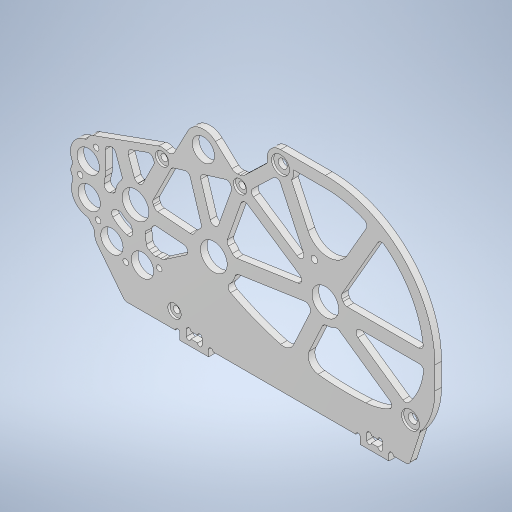
# Autodesk Inventor part: ギアマウント
Saved by Autodesk Inventor 2023 (Build 270158000, 158)
## iProperties
Created: 2022-03-20
Part Number: ギアマウント
Material: Aluminum 2014-T6
Document SubType Name: Modeling
Designer: acps
Density: 2.78927 g/cm^3
Appearance: Satin
Author: acps
Autodesk Inventor part; units mm, degrees
ref_plane "YZ Plane" through (0, 0, 0) normal (1, 0, 0) x (0, 1, 0)
ref_plane "XZ Plane" through (0, 0, 0) normal (0, 1, 0) x (-1, 0, 0)
ref_plane "XY Plane" through (0, 0, 0) normal (0, 0, 1) x (1, 0, 0)
sketch "Sketch2" plane through (0, 0, 0) normal (0, 0, 1) x (1, 0, 0)
  line L0 (-44.2416, -60) -> (63.0185, -60) construction
  line L1 (-44.2416, -60) -> (63.0185, -60) construction
  circle A0 centre (-30.6992, 12) radius 14 construction
  circle A1 centre (-44.5148, 14.4973) radius 14 construction
  circle A2 centre (-50.7402, 19.5218) radius 1.25
  circle A3 centre (-38.2895, 9.4728) radius 1.25
  circle A4 centre (-23.1088, 14.5272) radius 1.25
  circle A5 centre (-58.8465, 33.3162) radius 1.25
  circle A6 centre (-51.6122, 47.5873) radius 1.25
  circle A7 centre (-55.2294, 40.4518) radius 14 construction
  circle A8 centre (-54.7933, 26.419) radius 14 construction
  circle A9 centre (-33.8392, 34.0933) radius 22.3153 construction
  circle A10 centre (1.5644, 31.4) radius 30.9859 construction
  circle A11 centre (52, 38.9589) radius 41.9589 construction
  circle A12 centre (-55.2294, 40.4518) radius 5.025
  arc A13 (-56.8528, 48.3109) -> (-62.589, 43.6511) centre (-55.2294, 40.4518) ccw
  circle A14 centre (-54.7933, 26.419) radius 5.025
  circle A15 centre (-54.7933, 26.419) radius 8.025
  circle A16 centre (-50.7402, 19.5218) radius 4.25 construction
  arc A17 (-36.8441, 5.4762) -> (-41.0426, 6.2351) centre (-38.2895, 9.4728) ccw construction
  arc A18 (-24.5543, 18.5238) -> (-21.87, 10.4617) centre (-23.1088, 14.5272) ccw construction
  circle A19 centre (-44.5148, 14.4973) radius 5.025
  circle A20 centre (-30.6992, 12) radius 5.025
  circle A21 centre (-44.5148, 14.4973) radius 8.025
  circle A22 centre (-30.6992, 12) radius 8.025
  arc A23 (-41.0426, 6.2351) -> (-42.7724, 6.6637) centre (-42.3382, 4.7114) ccw
  arc A24 (-56.8528, 48.3109) -> (-55.451, 49.4112) centre (-57.2574, 50.2695) ccw
  arc A25 (-35.0737, 5.2721) -> (-36.8441, 5.4762) centre (-36.1639, 3.5954) ccw
  circle A26 centre (-21.8397, 58.0739) radius 1.5
  circle A27 centre (-21.8397, 58.0739) radius 4.5
  circle A28 centre (13.4218, 64.8462) radius 1.5
  circle A29 centre (13.4218, 64.8462) radius 4.5
  circle A30 centre (31.7211, 82.4471) radius 6.025
  circle A31 centre (31.7211, 82.4471) radius 4.025
  circle A32 centre (90.487, 12.01) radius 5.025
  circle A33 centre (90.487, 12.01) radius 2.025
  line L2 (-53.0558, 51.5846) -> (-23.3682, 62.3063)
  arc A34 (-18.3854, 60.958) -> (-16.2563, 60.33) centre (-16.8502, 62.2398) ccw
  line L3 (-16.2563, 60.33) -> (12.0856, 69.1432)
  circle A35 centre (-33.8392, 34.0933) radius 6.025
  circle A36 centre (-33.8392, 34.0933) radius 9.025
  arc A37 (-47.4788, 38.3562) -> (-31.6308, 19.9746) centre (-33.8392, 34.0933) ccw
  line L4 (-46.0723, 50.9171) -> (-28.4446, 57.2833)
  arc A38 (-25.942, 56.2243) -> (-28.4446, 57.2833) centre (-27.7652, 55.4023) ccw
  arc A39 (-25.6321, 53.8469) -> (-25.7034, 55.7671) centre (-27.4207, 54.7419) ccw
  line L5 (-25.6321, 53.8469) -> (-30.5023, 44.114)
  arc A40 (-32.5717, 43.0288) -> (-30.5023, 44.114) centre (-32.2908, 45.009) ccw
  line L6 (-17.8154, 56.0602) -> (-25.8299, 40.0433)
  arc A41 (-25.8299, 40.0433) -> (-25.8187, 38.2313) centre (-24.0414, 39.1483) ccw
  line L7 (-33.8392, 34.0933) -> (-21.8397, 58.0739) construction
  line L8 (-47.4788, 38.3562) -> (-47.4212, 38.5991)
  line L9 (-47.2048, 40.5594) -> (-47.3924, 48.9915)
  arc A42 (-46.0723, 50.9171) -> (-47.3924, 48.9915) centre (-45.3929, 49.036) ccw
  line L10 (-54.7933, 26.419) -> (-33.8392, 34.0933) construction
  arc A43 (-48.0965, 35.0629) -> (-45.4133, 33.0492) centre (-46.1011, 34.9272) ccw
  arc A44 (-43.3499, 27.4152) -> (-44.0979, 24.1448) centre (-42.6621, 25.5372) ccw
  arc A45 (-44.0976, 33.5311) -> (-42.7997, 35.1704) centre (-44.7854, 35.4091) ccw
  arc A46 (-39.9845, 27.4838) -> (-42.0342, 27.8971) centre (-41.3464, 26.019) ccw
  line L11 (-45.4133, 33.0492) -> (-44.0976, 33.5311)
  line L12 (-43.3499, 27.4152) -> (-42.0342, 27.8971)
  line L13 (-33.8392, 34.0933) -> (-30.6992, 12) construction
  arc A47 (-35.4267, 23.9429) -> (-36.7596, 25.5538) centre (-37.4068, 23.6614) ccw
  arc A48 (-28.6551, 26.7057) -> (-29.4864, 24.7871) centre (-27.5063, 25.0686) ccw
  arc A49 (-37.7581, 20.3508) -> (-35.2295, 22.5556) centre (-37.2096, 22.2742) ccw
  arc A50 (-28.9517, 21.0248) -> (-27.7152, 19.4496) centre (-26.9716, 21.3062) ccw
  line L14 (-35.4267, 23.9429) -> (-35.2295, 22.5556)
  line L15 (-29.4864, 24.7871) -> (-28.9517, 21.0248)
  arc A51 (-42.7678, 49.9841) -> (-45.3282, 51.1858) centre (-44.6489, 49.3047) ccw
  arc A52 (-35.9228, 54.5826) -> (-37.1245, 52.0221) centre (-35.2435, 52.7015) ccw
  arc A53 (-40.421, 40.2682) -> (-39.9985, 42.316) centre (-41.8796, 41.6367) ccw
  arc A54 (-34.3552, 44.3541) -> (-32.7218, 43.0488) centre (-32.4741, 45.0334) ccw
  line L16 (-42.7678, 49.9841) -> (-39.9985, 42.316)
  line L17 (-34.3552, 44.3541) -> (-37.1245, 52.0221)
  line L18 (-33.8392, 34.0933) -> (-40.6255, 52.8842) construction
  circle A55 centre (1.5644, 31.4) radius 6.025
  circle A56 centre (52, 38.9589) radius 6.025
  circle A57 centre (1.5644, 31.4) radius 10.025
  circle A58 centre (52, 38.9589) radius 9.025
  arc A59 (-16.6207, 57.075) -> (-17.8154, 56.0602) centre (-16.0268, 55.1652) ccw
  line L19 (-16.6207, 57.075) -> (6.788, 64.3542)
  arc A60 (9.2403, 63.1834) -> (6.788, 64.3542) centre (7.3818, 62.4444) ccw
  arc A61 (-26.3247, 18.7279) -> (-24.5543, 18.5238) centre (-25.2345, 20.4046) ccw
  arc A62 (-21.87, 10.4617) -> (-23.1648, 9.2372) centre (-21.287, 8.5486) ccw
  arc A63 (-22.4016, 18.7179) -> (-20.9398, 19.0391) centre (-22.0688, 20.69) ccw
  arc A64 (-18.1174, 14.9119) -> (-18.947, 13.6662) centre (-16.9884, 13.261) ccw
  line L20 (-20.9398, 19.0391) -> (-11.0791, 25.7824)
  arc A65 (-9.0516, 27.1689) -> (-8.2271, 29.249) centre (-10.1805, 28.8198) ccw construction
  arc A66 (-3.9917, 23.0555) -> (-6.2292, 23.0417) centre (-5.1002, 21.3908) ccw
  line L21 (-18.1174, 14.9119) -> (-6.2292, 23.0417)
  line L22 (-23.1088, 14.5272) -> (1.5644, 31.4) construction
  arc A67 (-25.5084, 37.5643) -> (-23.8139, 36.3393) centre (-23.6622, 38.3335) ccw
  arc A68 (-24.269, 30.3566) -> (-26.1293, 29.4019) centre (-24.4207, 28.3623) ccw
  arc A69 (-9.1127, 35.2209) -> (-7.2104, 36.248) centre (-8.961, 37.2151) ccw
  arc A70 (-7.8428, 27.9352) -> (-9.5679, 29.2382) centre (-9.7196, 27.244) ccw construction
  line L23 (-23.8139, 36.3393) -> (-9.1127, 35.2209)
  line L24 (-24.269, 30.3566) -> (-12.0564, 29.4275)
  line L25 (-33.8392, 34.0933) -> (1.5644, 31.4) construction
  arc A71 (-11.0791, 25.7824) -> (-12.0564, 29.4275) centre (-12.2081, 27.4333) ccw
  line L26 (-12.0564, 29.4275) -> (-9.5679, 29.2382) construction
  line L27 (-11.0791, 25.7824) -> (-9.0516, 27.1689) construction
  line L28 (-7.319, 59.9675) -> (1.5644, 31.4) construction
  arc A72 (-9.1123, 57.3153) -> (-11.616, 58.6313) centre (-11.0221, 56.7215) ccw
  arc A73 (-3.0219, 61.3037) -> (-4.3379, 58.8) centre (-2.4281, 59.3939) ccw
  arc A74 (-4.7785, 39.1633) -> (-4.2408, 41.5776) centre (-6.0439, 40.7121) ccw
  arc A75 (0.6404, 42.7907) -> (2.3863, 41.3913) centre (2.5502, 43.3845) ccw construction
  line L29 (-9.1123, 57.3153) -> (-4.1341, 41.306)
  line L30 (-4.3379, 58.8) -> (-0.0658, 45.0619)
  arc A76 (-55.451, 49.4112) -> (-55.772, 48.4584) centre (-51.6122, 47.5873) ccw construction
  arc A77 (-55.772, 48.4584) -> (-56.8528, 48.3109) centre (-55.2294, 40.4518) ccw construction
  arc A78 (-62.589, 43.6511) -> (-62.0081, 36.1565) centre (-55.2294, 40.4518) ccw
  arc A79 (-62.0081, 36.1565) -> (-55.772, 48.4584) centre (-55.2294, 40.4518) ccw
  arc A80 (-53.0558, 51.5846) -> (-55.451, 49.4112) centre (-51.6122, 47.5873) ccw
  arc A81 (-41.0426, 6.2351) -> (-36.8441, 5.4762) centre (-38.2895, 9.4728) ccw
  arc A82 (-22.4016, 18.7179) -> (-24.5543, 18.5238) centre (-23.1088, 14.5272) ccw
  arc A83 (-18.947, 13.6662) -> (-22.4016, 18.7179) centre (-23.1088, 14.5272) ccw construction
  arc A84 (-21.4252, 10.6249) -> (-18.947, 13.6662) centre (-23.1088, 14.5272) ccw
  arc A85 (-21.87, 10.4617) -> (-21.4252, 10.6249) centre (-23.1088, 14.5272) ccw
  arc A86 (9.9632, 36.8737) -> (11.9352, 35.9878) centre (11.6387, 37.9657) ccw
  arc A87 (12.8245, 30.0541) -> (11.1988, 28.629) centre (13.1209, 28.0762) ccw
  arc A88 (41.8379, 40.4694) -> (43.4387, 41.8145) centre (41.5414, 42.4473) ccw construction
  arc A89 (44.652, 33.7189) -> (42.7272, 34.5357) centre (43.0236, 32.5577) ccw
  line L31 (11.9352, 35.9878) -> (39.536, 40.1244)
  line L32 (12.8245, 30.0541) -> (42.7272, 34.5357)
  line L33 (1.5644, 31.4) -> (52, 38.9589) construction
  arc A90 (9.4982, 61.2607) -> (9.4005, 62.8266) centre (7.6132, 61.929) ccw
  arc A91 (15.2731, 60.7446) -> (14.2108, 59.59) centre (16.0959, 58.9217) ccw construction
  arc A92 (1.1349, 41.4158) -> (2.9342, 42.7457) centre (1.0492, 43.414) ccw construction
  arc A93 (7.6468, 41.0749) -> (8.2067, 38.9087) centre (9.5319, 40.4067) ccw
  line L34 (2.9342, 42.7457) -> (3.729, 44.9875) construction
  line L35 (14.2108, 59.59) -> (13.8416, 58.5486) construction
  line L36 (1.5644, 31.4) -> (13.4218, 64.8462) construction
  arc A94 (-0.0658, 45.0619) -> (3.729, 44.9875) centre (1.844, 45.6558) ccw
  line L37 (-0.0658, 45.0619) -> (0.6404, 42.7907) construction
  line L38 (3.729, 44.9875) -> (9.4982, 61.2607)
  line L39 (13.4218, 64.8462) -> (52, 38.9589) construction
  arc A95 (15.9236, 60.1567) -> (14.3823, 60.4499) centre (14.8092, 58.496) ccw construction
  arc A96 (17.8541, 65.6237) -> (18.7096, 64.3086) centre (19.824, 65.9693) ccw construction
  arc A97 (43.106, 40.4909) -> (42.2494, 42.4912) centre (41.135, 40.8304) ccw construction
  arc A98 (45.0355, 46.643) -> (47.2111, 46.6086) centre (46.1499, 48.3038) ccw construction
  line L40 (18.7096, 64.3086) -> (19.45, 63.8118) construction
  line L41 (42.2494, 42.4912) -> (40.354, 43.7631) construction
  arc A99 (16.8411, 59.541) -> (13.8416, 58.5486) centre (15.7267, 57.8803) ccw
  line L42 (13.8416, 58.5486) -> (7.6468, 41.0749)
  line L43 (16.8411, 59.541) -> (15.9236, 60.1567) construction
  arc A100 (39.536, 40.1244) -> (40.354, 43.7631) centre (39.2396, 42.1023) ccw
  line L44 (40.354, 43.7631) -> (16.8411, 59.541)
  line L45 (39.536, 40.1244) -> (41.8379, 40.4694) construction
  line L46 (31.7211, 82.4471) -> (52, 38.9589) construction
  line L47 (52, 38.9589) -> (90.487, 12.01) construction
  line L48 (52, 38.9589) -> (96.5132, 38.9589) construction
  arc A101 (-3.9917, 23.0555) -> (91.7705, 7.1517) centre (61.5599, 121.5041) ccw
  arc A102 (9.1166, 21.0995) -> (70.407, 8.5744) centre (61.5599, 121.5041) ccw
  arc A103 (8.6324, 24.2906) -> (9.1166, 21.0995) centre (10.0425, 22.8723) ccw
  arc A104 (45.1595, 31.2935) -> (44.9138, 33.3699) centre (43.3435, 32.1314) ccw
  arc A105 (52.3468, 29.9406) -> (50.6076, 28.7799) centre (52.4236, 27.942) ccw
  line L49 (45.1595, 31.2935) -> (37.6177, 14.9471)
  line L50 (50.6076, 28.7799) -> (44.7222, 16.0237)
  arc A106 (31.7623, 12.2178) -> (37.6177, 14.9471) centre (33.0776, 17.0418) ccw
  arc A107 (44.7222, 16.0237) -> (48.6944, 8.9614) centre (49.2623, 13.929) ccw
  line L51 (38.88, 10.5221) -> (52, 38.9589) construction
  arc A108 (13.6025, 69.3426) -> (15.0693, 69.8995) centre (13.6828, 71.341) ccw
  arc A109 (18.5354, 66.2959) -> (17.9218, 64.8519) centre (19.9218, 64.8544) ccw construction
  line L52 (15.0693, 69.8995) -> (25.1991, 79.6427)
  arc A110 (25.1991, 79.6427) -> (25.7837, 81.4239) centre (23.8127, 81.0842) ccw
  arc A111 (30.4677, 76.5539) -> (28.6652, 76.0391) centre (30.0517, 74.5976) ccw construction
  line L53 (18.5354, 66.2959) -> (19.178, 66.914) construction
  line L54 (13.4218, 64.8462) -> (31.7211, 82.4471) construction
  arc A112 (19.178, 66.914) -> (19.45, 63.8118) centre (20.5644, 65.4725) ccw
  line L55 (19.178, 66.914) -> (28.536, 75.9148)
  line L56 (19.45, 63.8118) -> (39.1784, 50.5734)
  arc A113 (31.655, 75.4903) -> (30.3106, 76.5895) centre (29.8424, 74.6451) ccw construction
  arc A114 (44.8912, 44.519) -> (45.1284, 46.5964) centre (43.3158, 45.7512) ccw construction
  line L57 (45.1284, 46.5964) -> (42.1054, 53.0793) construction
  arc A115 (37.115, 79.7624) -> (37.0928, 78.026) centre (38.9054, 78.8713) ccw construction
  line L58 (44.165, 62.8598) -> (35.8801, 80.6268)
  arc A116 (31.7351, 75.3186) -> (28.536, 75.9148) centre (29.9224, 74.4734) ccw
  line L59 (28.536, 75.9148) -> (28.6652, 76.0391) construction
  line L60 (31.7351, 75.3186) -> (31.655, 75.4903) construction
  arc A117 (39.1784, 50.5734) -> (42.1054, 53.0793) centre (40.2928, 52.2341) ccw
  line L61 (42.1054, 53.0793) -> (31.7351, 75.3186)
  line L62 (39.1784, 50.5734) -> (45.0355, 46.643) construction
  arc A118 (101.5132, 38.9589) -> (52, 88.4721) centre (52, 38.9589) ccw
  arc A119 (39.6867, 83.4721) -> (37.7015, 81.7151) centre (39.6867, 81.4721) ccw construction
  line L63 (31.7211, 88.4721) -> (52, 88.4721)
  line L64 (39.6867, 83.4721) -> (37.6927, 83.4721) construction
  arc A120 (37.6927, 83.4721) -> (35.8801, 80.6268) centre (37.6927, 81.4721) ccw
  line L65 (37.6927, 83.4721) -> (52, 83.4721)
  line L66 (35.8801, 80.6268) -> (37.0928, 78.026) construction
  arc A121 (96.5132, 38.9589) -> (52, 83.4721) centre (52, 38.9589) ccw
  line L67 (96.5132, 38.9589) -> (96.5132, 36.8058)
  line L68 (101.5132, 38.9589) -> (101.5132, 28.7597)
  arc A122 (94.3686, 8.8189) -> (101.5132, 28.7597) centre (70.1132, 28.7597) ccw
  arc A123 (70.407, 8.5744) -> (96.5132, 36.8058) centre (68.1953, 36.8058) ccw
  arc A124 (58.3283, 30.8655) -> (56.2412, 30.9926) centre (57.1811, 29.2272) ccw
  arc A125 (60.9365, 37.6981) -> (61.7697, 35.7804) centre (62.9169, 37.4187) ccw
  arc A126 (80.866, 11.4808) -> (81.1183, 14.9077) centre (79.9711, 13.2694) ccw
  arc A127 (87.0584, 18.0731) -> (89.7262, 18.4123) centre (88.2056, 19.7114) ccw
  line L69 (58.3283, 30.8655) -> (81.1183, 14.9077)
  line L70 (61.7697, 35.7804) -> (87.0584, 18.0731)
  line L71 (52, 38.9589) -> (74.2566, 77.5084) construction
  arc A128 (59.5111, 45.9685) -> (59.5664, 43.8783) centre (61.2431, 44.9685) ccw
  arc A129 (70.511, 77.0209) -> (69.5683, 79.8585) centre (68.7789, 78.0209) ccw
  arc A130 (78.636, 74.6233) -> (75.7071, 74.0209) centre (77.4392, 73.0209) ccw
  line L72 (70.511, 77.0209) -> (61.8883, 62.0859)
  line L73 (59.5111, 45.9685) -> (75.7071, 74.0209)
  line L74 (61.826, 41.9589) -> (94.2181, 41.9589)
  line L75 (67.858, 35.9589) -> (94.5132, 35.9589)
  arc A131 (67.858, 35.9589) -> (66.7108, 32.3206) centre (67.858, 33.9589) ccw
  arc A132 (60.0435, 43.0519) -> (61.826, 41.9589) centre (61.826, 43.9589) ccw
  arc A133 (94.2181, 41.9589) -> (96.2042, 44.1941) centre (94.2181, 43.9589) ccw
  arc A134 (96.5132, 33.9589) -> (94.5132, 35.9589) centre (94.5132, 33.9589) ccw
  arc A135 (-39.285, -5.2313) -> (-37.709, -6) centre (-37.709, -4) ccw
  line L76 (-33.8392, 34.0933) -> (-16.1374, 34.0933) construction
  line L77 (1.5644, 34.0933) -> (1.5644, 31.4) construction
  line L78 (-16.1374, 34.0933) -> (-16.1374, 29.0871) construction
  arc A136 (88.4657, -6) -> (90.3678, -4.618) centre (88.4657, -4) ccw
  arc A137 (-62.5868, 35.3343) -> (-62.528, 37.1155) centre (-64.347, 36.284) ccw
  arc A138 (-62.5868, 35.3343) -> (-62.4543, 31.0698) centre (-58.8465, 33.3162) ccw
  arc A139 (-62.285, 29.2957) -> (-62.4543, 31.0698) centre (-64.1521, 30.0127) ccw
  line L79 (-37.709, -6) -> (88.4657, -6)
  line L80 (-10.7865, -3) -> (77.7566, -3)
  circle A140 centre (-9.7865, -3) radius 1
  circle A141 centre (-4.7865, -3) radius 1
  circle A142 centre (-9.7865, -6) radius 1
  circle A143 centre (-4.7865, -6) radius 1
  line L81 (-10.7865, -3) -> (-10.7865, -6)
  line L82 (-3.7865, -3) -> (-3.7865, -6)
  circle A144 centre (-14.7865, -6) radius 1
  circle A145 centre (0.2135, -6) radius 1
  circle A146 centre (71.7566, -3) radius 1
  circle A147 centre (76.7566, -3) radius 1
  circle A148 centre (71.7566, -6) radius 1
  circle A149 centre (76.7566, -6) radius 1
  line L83 (77.7566, -3) -> (77.7566, -6)
  line L84 (70.7566, -3) -> (70.7566, -6)
  circle A150 centre (66.7566, -6) radius 1
  circle A151 centre (81.7566, -6) radius 1
  line L85 (-13.7865, -6) -> (-13.7865, -9)
  line L86 (-13.7865, -9) -> (-0.7865, -9)
  line L87 (-0.7865, -9) -> (-0.7865, -6)
  line L88 (67.7566, -6) -> (67.7566, -9)
  line L89 (67.7566, -9) -> (80.7566, -9)
  line L90 (80.7566, -9) -> (80.7566, -6)
  circle A152 centre (-16.2379, 1.2821) radius 1.5
  circle A153 centre (-16.2379, 1.2821) radius 3
  circle A154 centre (-16.2379, 1.2821) radius 4 construction
  arc A155 (-54.4583, 17.4631) -> (-55.9258, 18.4743) centre (-56.208, 16.4943) ccw
  arc A156 (-54.4583, 17.4631) -> (-53.3238, 16.1473) centre (-50.7402, 19.5218) ccw
  arc A157 (-52.5397, 14.5469) -> (-53.3238, 16.1473) centre (-54.5396, 14.5593) ccw
  line L91 (-39.285, -5.2313) -> (-50.8386, 9.5566)
  line L92 (-16.1374, 34.0933) -> (1.5644, 34.0933) construction
  line L93 (-7.2865, 34.0933) -> (-7.2865, -12.1424) construction
  circle A158 centre (-21.8397, 58.0739) radius 3
  circle A159 centre (13.4218, 64.8462) radius 3
  circle A160 centre (-3.14, 71) radius 5.025
  circle A161 centre (-3.14, 71) radius 8.025
  line L94 (-10.2436, 74.7336) -> (-16.1326, 63.5293)
  arc A162 (-20.0087, 62.1846) -> (-16.1326, 63.5293) centre (-18.7881, 64.925) ccw
  line L95 (2.3049, 76.8952) -> (9.7999, 69.9727)
  arc A163 (9.7999, 69.9727) -> (12.4699, 69.2444) centre (11.8354, 72.1765) ccw
  line L96 (95.266, 10.4572) -> (90.3678, -4.618)
  line L97 (74.2566, 38.9589) -> (74.2566, -10.9885) construction
  circle A164 centre (31.7211, 82.4471) radius 2.025
  circle A165 centre (47, 53.101) radius 1.5
  arc A166 (44.165, 62.8598) -> (61.8883, 62.0859) centre (53.2281, 67.0859) ccw
  circle A167 centre (90.487, 12.01) radius 4.025
  point P0 (0, 0)
  point P1 (-47.2064, 40.6303)
  point P2 (-47.537, 38.1651)
  point P3 (96.4233, 34.5517)
  point P4 (36.6482, 78.9795)
  point P5 (37.6584, 83.4718)
  point P6 (72.7566, -3)
  point P7 (75.7566, -3)
  point P8 (75.7566, -6)
  point P9 (72.7566, -6)
  point P10 (-5.7865, -6)
  point P11 (-8.7865, -6)
  point P12 (-8.7865, -3)
  point P13 (-5.7865, -3)
  point P14 (-15.7865, -6)
  point P15 (1.2135, -6)
  point P16 (65.7566, -6)
  point P17 (82.7566, -6)
  point P18 (94.9855, 9.5939)
  dimension "d1136" = 2
  dimension "d1137" = 2
  dimension "d1139" = 2
  dimension "d1140" = 2
  dimension "d1142" = 2
  dimension "d1144" = 2
  dimension "d1146" = 2
  dimension "d1147" = 2
  dimension "d1149" = 2
  dimension "d1150" = 2
  dimension "d1152" = 2
  dimension "d1153" = 2
  dimension "d984" = 60
  dimension "d985" = 10.05
  dimension "d986" = 3
  dimension "d987" = 10.05
  dimension "d988" = 3
  dimension "d989" = 3
  dimension "d990" = 3
  dimension "d991" = 3
  dimension "d992" = 10.05
  dimension "d993" = 10.05
  dimension "d994" = 3
  dimension "d995" = 3
  dimension "d996" = 2
  dimension "d997" = 2
  dimension "d998" = 2
  dimension "d999" = 3
  dimension "d1000" = 3
  dimension "d1001" = 3
  dimension "d1002" = 3
  dimension "d1003" = 8.05
  dimension "d1004" = 2
  dimension "d1005" = 4.05
  dimension "d1006" = 3
  dimension "d1007" = 2
  dimension "d1008" = 12.05
  dimension "d1009" = 3
  dimension "d1010" = 2
  dimension "d1011" = 3
  dimension "d1012" = 2
  dimension "d1013" = 2
  dimension "d1014" = 2
  dimension "d1015" = 6
  dimension "d1016" = 2
  dimension "d1017" = 2
  dimension "d1018" = 2
  dimension "d1019" = 2
  dimension "d1020" = 2
  dimension "d1021" = 3
  dimension "d1022" = 6
  dimension "d1023" = 2
  dimension "d1024" = 2
  dimension "d1025" = 2
  dimension "d1026" = 2
  dimension "d1027" = 6
  dimension "d1028" = 3
  dimension "d1029" = 2
  dimension "d1030" = 2
  dimension "d1031" = 2
  dimension "d1032" = 2
  dimension "d1033" = 6
  dimension "d1034" = 3
  dimension "d1035" = 12.05
  dimension "d1036" = 12.05
  dimension "d1037" = 4
  dimension "d1038" = 3
  dimension "d1039" = 2
  dimension "d1040" = 2
  dimension "d1041" = 3
  dimension "d1042" = 2
  dimension "d1043" = 2
  dimension "d1044" = 2
  dimension "d1045" = 2
  dimension "d1046" = 2
  dimension "d1047" = 2
  constraints: 266 point on circle, 217 tangent, 194 end point, 148 centre point, 60 parallel, 14 point on line, 14 vertical, 13 coincident, 9 horizontal, 7 perpendicular, 5 concentric, 2 midpoint, 192 other
  measures "d984" distance from line of L1 point (0, 0)
  measures "d985" diameter of A12
  measures "d987" diameter of A14
  measures "d988" radial gap between concentric circles of A14 A15
  measures "d989" radial gap between concentric circles of A2 A16
  measures "d990" radial gap between concentric circles of A3 A17
  measures "d991" radial gap between concentric circles of A4 A18
  measures "d992" diameter of A19
  measures "d993" diameter of A20
  measures "d994" radial gap between concentric circles of A19 A21
  measures "d995" radial gap between concentric circles of A20 A22
  measures "d996" radius of A24
  measures "d997" radius of A23
  measures "d998" radius of A25
  measures "d999" diameter of A26
  measures "d1000" radial gap between concentric circles of A26 A27
  measures "d1001" diameter of A28
  measures "d1002" diameter of A28
  measures "d1003" diameter of A31
  measures "d1004" radial gap between concentric circles of A31 A30
  measures "d1005" diameter of A33
  measures "d1006" radial gap between concentric circles of A33 A32
  measures "d1007" radius of A34
  measures "d1008" diameter of A35
  measures "d1010" radius of A38
  measures "d1011" distance between parallel lines of L2 L4
  measures "d1012" radius of A39
  measures "d1013" radius of A40
  measures "d1014" radius of A41
  measures "d1015" distance between parallel lines of L5 L6
  measures "d1016" radius of A42
  measures "d1017" radius of A43
  measures "d1018" radius of A44
  measures "d1019" radius of A45
  measures "d1020" radius of A46
  measures "d1021" distance between parallel lines of L11 L10
  measures "d1022" distance between parallel lines of L12 L11
  measures "d1023" radius of A47
  measures "d1024" radius of A48
  measures "d1025" radius of A49
  measures "d1026" radius of A50
  measures "d1027" distance between parallel lines of L15 L14
  measures "d1028" distance between parallel lines of L14 L13
  measures "d1029" radius of A51
  measures "d1030" radius of A52
  measures "d1031" radius of A53
  measures "d1032" radius of A54
  measures "d1033" distance between parallel lines of L17 L16
  measures "d1034" distance between parallel lines of L16 L18
  measures "d1035" diameter of A55
  measures "d1036" diameter of A56
  measures "d1039" radius of A59
  measures "d1040" radius of A60
  measures "d1041" distance between parallel lines of L19 L3
  measures "d1042" radius of A61
  measures "d1043" radius of A62
  measures "d1044" radius of A63
  measures "d1045" radius of A64
  measures "d1046" radius of A65
  measures "d1047" radius of A66
extrude "Extrusion1" add sketch "Sketch2" along normal blind 3 contours A2 A15 A21 A22 A3 | A2 A21 A15 | A21 A157 A156 A155 A15 A2 | A2 A15 A5 A79 A21 | A15 A37 A21 | A37 A22 A21 | A21 A23 A81 A25 A22 A62 A85 A84 A64 L21 A66 A101 A32 A122 L96 A136 L79 A151 L83 A147 L80 A146 A141 A140 L81 A144 A135 L91 | A15 A79 A37 | A37 A43 L11 A45 A36 A46 L12 A44 | A22 A4 A3 A21 | A21 A3 A22 | A49 L14 A47 A36 A48 L15 A50 A22 A37 | A139 A138 A137 A78 A79 A5 A15 | A21 A3 A22 A25 A81 A23 | A79 A5 A15 | A15 A5 A79 A78 A13 A24 A80 L2 A27 A38 L4 A42 L9 | A61 A82 A63 L20 A71 L24 A68 A36 A67 L23 A69 A57 A66 L21 A64 A84 A85 A62 A22 A4 | A36 | L79 A142 A143 L87 L86 L85 | A53 L16 A51 L4 A52 L17 A54 A36 | L79 L82 L80 L84 A150 A145 | A40 L5 A39 A27 L6 A41 A36 | A27 | A162 L94 A161 L3 A34 A27 | L79 A148 A149 L90 L89 L88 | A27 A34 L3 A161 A29 A60 L19 A59 | A57 | A57 A103 A102 A123 A32 A101 | A74 L29 A72 L19 A73 L30 A94 L38 A90 A29 A108 L52 A110 A30 L58 A166 L72 A129 A121 A130 L73 A128 A58 A89 L32 A87 A57 A86 L31 A100 L44 A99 L42 A93 | A161 L3 | A32 | L3 A161 | L95 A163 A29 L3 A161 | A123 L67 A121 L65 A120 A30 L63 A118 L68 A122 L96 A32 | A123 A126 L69 A124 A58 A125 L70 A127 | A106 L49 A104 A58 A105 L50 A107 A102 | A29 | A134 L75 A131 L70 A125 A58 A132 L74 A133 A121 L67 A123 | A58 | A30 A120 L58 | A30 L58 A120 picked at (-49.1846, 20.8215) picked at (-37.9272, 13.1818) picked at (-54.9204, 33.1261)
extrude "Extrusion2" add sketch "Sketch2" along normal blind 2 contours A31 | A153 | A158 | A159 | A167
body "Solid1"
